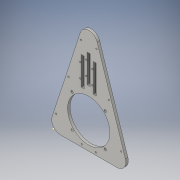
# Autodesk Inventor part: Nathan_LED_Speaker_Front
Saved by Autodesk Inventor 2016 (Build 200138000, 138)
## iProperties
Created: 2018-09-27
Part Number: Nathan_LED_Speaker_Front
Material: Generic
Document SubType Name: Modeling
Designer: Student
Density: 1 g/cm^3
Appearance: Default
Author: Student
Autodesk Inventor part; units mm, degrees
ref_plane "YZ Plane" through (0, 0, 0) normal (1, 0, 0) x (0, 1, 0)
ref_plane "XZ Plane" through (0, 0, 0) normal (0, 1, 0) x (-1, 0, 0)
ref_plane "XY Plane" through (0, 0, 0) normal (0, 0, 1) x (1, 0, 0)
sketch "Sketch1" plane through (0, 0, 0) normal (0, 0, 1) x (1, 0, 0)
  line L0 (63.5, 50.8) -> (63.5, 44.45)
  circle A0 centre (63.5, 44.45) radius 38.1
  circle A1 centre (33.655, 74.295) radius 2.1082
  circle A2 centre (93.345, 74.295) radius 2.1082
  circle A3 centre (93.345, 14.605) radius 2.1082
  circle A4 centre (33.655, 14.605) radius 2.1082
  line L1 (63.5, 82.55) -> (63.5, 86.36)
  line L2 (63.5, 86.36) -> (82.55, 86.36)
  line L3 (63.5, 86.36) -> (44.45, 86.36)
  line L4 (82.55, 86.36) -> (82.55, 134.62)
  line L5 (44.45, 86.36) -> (44.45, 134.62)
  arc A5 (82.55, 134.62) -> (44.45, 134.62) centre (63.5, 134.62) ccw
  arc A6 (-2.400661, 17.597517) -> (12.7, -3.175) centre (12.7, 12.7) ccw
  arc A7 (114.3, -3.175) -> (129.400661, 17.597517) centre (114.3, 12.7) ccw
  line L6 (114.3, -3.175) -> (12.7, -3.175)
  line L7 (48.399339, 174.230681) -> (-2.400661, 17.597517)
  line L8 (129.400661, 17.597517) -> (78.600661, 174.230681)
  arc A8 (78.600661, 174.230681) -> (48.399339, 174.230681) centre (63.5, 169.333164) ccw
  arc A9 (75.580529, 173.251177) -> (51.419471, 173.251177) centre (63.5, 169.333164) ccw
  arc A10 (0.619471, 16.618013) -> (12.7, 0) centre (12.7, 12.7) ccw
  arc A11 (114.3, 0) -> (126.380529, 16.618013) centre (114.3, 12.7) ccw
  line L9 (12.7, 0) -> (114.3, 0)
  line L10 (0.619471, 16.618013) -> (51.419471, 173.251177)
  line L11 (75.580529, 173.251177) -> (126.380529, 16.618013)
  line L12 (0.619471, 16.618013) -> (3.753882, 26.282436)
  line L13 (3.753882, 26.282436) -> (4.961935, 25.890635)
  circle A12 centre (4.961935, 25.890635) radius 1.27
  line L14 (51.419471, 173.251177) -> (48.285061, 163.586755)
  line L15 (48.285061, 163.586755) -> (49.493113, 163.194953)
  circle A13 centre (49.493113, 163.194953) radius 1.27
  circle A14 centre (27.227524, 94.542794) radius 1.27
  line L16 (75.580529, 173.251177) -> (78.714939, 163.586755)
  line L17 (78.714939, 163.586755) -> (77.506886, 163.194953)
  circle A15 centre (77.506886, 163.194953) radius 1.27
  line L18 (126.380529, 16.618013) -> (123.246118, 26.282436)
  line L19 (123.246118, 26.282436) -> (122.038065, 25.890635)
  circle A16 centre (122.038065, 25.890635) radius 1.27
  circle A17 centre (99.772476, 94.542794) radius 1.27
  line L20 (12.7, 0) -> (16.51, 0)
  line L21 (18.621315, -3.175) -> (18.621315, 1.27) construction
  line L22 (45.72, 1.27) -> (50.8, 1.27) construction
  line L23 (12.7, 0.808162) -> (16.51, 0.808162) construction
  circle A18 centre (50.8, 1.27) radius 1.27
  line L24 (109.391635, -3.175) -> (109.391635, 1.27) construction
  line L25 (81.28, 1.27) -> (76.2, 1.27) construction
  line L26 (114.432893, 0.578481) -> (110.622893, 0.578481) construction
  circle A19 centre (76.2, 1.27) radius 1.27
  point P0 (0, 0)
  point P1 (0, 0)
  dimension "d13" = 76.2
  dimension "d42" = 2.54
  dimension "d45" = 2.54
  dimension "d12" = 6.35
  dimension "d14" = 4.2164
  dimension "d15" = 4.2164
  dimension "d16" = 4.2164
  dimension "d17" = 4.2164
  dimension "d18" = 3.81
  dimension "d19" = 19.05
  dimension "d20" = 19.05
  dimension "d21" = 48.26
  dimension "d22" = 48.26
  dimension "d26" = 31.75
  dimension "d27" = 31.75
  dimension "d30" = 25.4
  dimension "d31" = 25.4
  dimension "d32" = 25.4
  dimension "d33" = 10.16
  dimension "d34" = 10.16
  dimension "d35" = 1.27
  dimension "d37" = 1.27
  dimension "d40" = 10.16
  dimension "d41" = 10.16
  dimension "d43" = 2.54
  dimension "d44" = 2.54
  dimension "d221" = 4.445
  dimension "d222" = 5.08
  dimension "d224" = 5.08
  dimension "d225" = 3.81
  dimension "d228" = 38.1
  dimension "d229" = 38.1
  constraints: 54 end point, 15 centre point, 14 point on circle, 10 coincident, 7 point on line, 6 horizontal, 6 tangent, 6 vertical, 1 perpendicular, 1 vertical alignment, 14 other
  measures "d12" distance of L0.start L0.end
  measures "d14" diameter of A1
  measures "d15" diameter of A2
  measures "d16" diameter of A3
  measures "d17" diameter of A4
  measures "d18" distance of L1.start L1.end
  measures "d19" distance of L1.end L2.end
  measures "d20" distance of L1.end L3.end
  measures "d21" distance of L2.end L4.end
  measures "d22" distance of L3.end L5.end
  measures "d26" diameter of A6
  measures "d27" diameter of A7
  measures "d30" diameter of A9
  measures "d31" diameter of A10
  measures "d32" diameter of A11
  measures "d33" distance of L10.start L12.end
  measures "d34" distance of L10.end L14.end
  measures "d35" distance of L14.end L15.end
  measures "d37" distance of L16.end L17.end
  measures "d40" distance of L11.end L18.end
  measures "d41" distance of L16.end L11.start
  measures "d43" diameter of A14
  measures "d44" diameter of A17
  measures "d221" distance of L21.start L21.end
  measures "d222" distance of L22.start L22.end
  measures "d224" distance of L25.start L25.end
  measures "d225" distance of L26.start L26.end
  measures "d228" horizontal distance of L25.end L6.start
  measures "d229" horizontal distance of L22.end L6.end
sketch "Sketch1 outline for Extrusion3" plane through (0, 0, 0) normal (0, 0, 1) x (1, 0, 0)
  arc A0 (78.600661, 174.230681) -> (48.399339, 174.230681) centre (63.5, 169.333164) ccw
  line L0 (129.400661, 17.597517) -> (78.600661, 174.230681)
  line L1 (48.399339, 174.230681) -> (-2.400661, 17.597517)
  arc A1 (114.3, -3.175) -> (129.400661, 17.597517) centre (114.3, 12.7) ccw
  arc A2 (-2.400661, 17.597517) -> (12.7, -3.175) centre (12.7, 12.7) ccw
  line L2 (12.7, -3.175) -> (114.3, -3.175)
  circle A3 centre (4.961935, 25.890635) radius 1.27
  circle A4 centre (33.655, 14.605) radius 2.1082
  circle A5 centre (33.655, 74.295) radius 2.1082
  circle A6 centre (93.345, 14.605) radius 2.1082
  circle A7 centre (63.5, 44.45) radius 38.1
  circle A8 centre (122.038065, 25.890635) radius 1.27
  circle A9 centre (93.345, 74.295) radius 2.1082
  circle A10 centre (27.227524, 94.542794) radius 1.27
  circle A11 centre (49.493113, 163.194953) radius 1.27
  line L3 (44.45, 86.36) -> (63.5, 86.36)
  line L4 (63.5, 86.36) -> (82.55, 86.36)
  line L5 (82.55, 86.36) -> (82.55, 134.62)
  arc A12 (82.55, 134.62) -> (44.45, 134.62) centre (63.5, 134.62) ccw
  line L6 (44.45, 134.62) -> (44.45, 86.36)
  circle A13 centre (99.772476, 94.542794) radius 1.27
  circle A14 centre (77.506886, 163.194953) radius 1.27
extrude "Extrusion3" add sketch "Sketch1 outline for Extrusion3" along normal blind 4.572
sketch "Sketch2" plane through (0, 0, 4.572) normal (0, 0, 1) x (1, 0, 0)
  line L0 (44.45, 86.36) -> (82.55, 86.36)
  line L1 (63.5, 86.36) -> (44.45, 86.36)
  line L2 (63.5, 86.36) -> (82.55, 86.36)
  line L3 (53.975, 86.36) -> (63.5, 86.36)
  line L4 (63.5, 86.36) -> (73.025, 86.36)
  line L5 (82.55, 134.62) -> (82.55, 86.36)
  line L6 (71.882, 140.7922) -> (76.962, 140.7922)
  line L7 (76.962, 140.7922) -> (76.962, 89.9922)
  line L8 (76.962, 89.9922) -> (71.882, 89.9922)
  line L9 (71.882, 89.9922) -> (71.882, 140.7922)
  circle A0 centre (70.07225, 128.0922) radius 1.3335
  circle A1 centre (70.07225, 102.6922) radius 1.3335
  line L10 (50.038, 89.9922) -> (55.118, 89.9922)
  line L11 (55.118, 89.9922) -> (55.118, 140.7922)
  line L12 (55.118, 140.7922) -> (50.038, 140.7922)
  line L13 (50.038, 140.7922) -> (50.038, 89.9922)
  line L14 (44.45, 86.36) -> (44.45, 134.62)
  circle A2 centre (48.22825, 128.0922) radius 1.3335
  circle A3 centre (48.22825, 102.6922) radius 1.3335
  line L15 (71.882, 99.06) -> (68.73875, 99.06)
  line L16 (66.04, 99.06) -> (60.96, 99.06)
  line L17 (60.96, 99.06) -> (60.96, 149.86)
  line L18 (60.96, 149.86) -> (66.04, 149.86)
  line L19 (66.04, 149.86) -> (66.04, 99.06)
  circle A4 centre (59.15025, 111.76) radius 1.3335
  circle A5 centre (59.15025, 137.16) radius 1.3335
  arc A6 (82.55, 134.62) -> (44.45, 134.62) centre (63.5, 134.62) ccw
  line L20 (44.45, 134.62) -> (44.45, 86.36)
  point P0 (0, 0)
  dimension "d183" = 5.08
  dimension "d184" = 50.8
  dimension "d185" = 3.6322
  dimension "d186" = 5.588
  dimension "d189" = 2.667
  dimension "d194" = 5.08
  dimension "d196" = 3.6322
  dimension "d197" = 5.588
  dimension "d198" = 50.8
  dimension "d199" = 1.80975
  dimension "d203" = 2.667
  dimension "d204" = 2.667
  dimension "d205" = 1.80975
  dimension "d207" = 41.7322
  dimension "d208" = 16.3322
  dimension "d209" = 1.80975
  dimension "d211" = 5.08
  dimension "d212" = 50.8
  dimension "d216" = 2.667
  dimension "d217" = 2.667
  constraints: 39 end point, 7 centre point, 6 horizontal, 6 parallel, 3 collinear, 3 midpoint, 3 perpendicular, 2 point on circle, 2 point on line, 1 vertical
  measures "d183" distance of L7.end L8.end
  measures "d184" distance of L6.end L7.end
  measures "d185" distance between parallel lines of L2 L8
  measures "d186" distance between parallel lines of L5 L7
  measures "d189" diameter of A0
  measures "d194" distance of L12.end L11.end
  measures "d196" distance between parallel lines of L1 L10
  measures "d197" distance between parallel lines of L14 L13
  measures "d198" distance of L12.end L10.start
  measures "d199" distance from line of L9 A1.centre
  measures "d203" diameter of A2
  measures "d204" diameter of A3
  measures "d205" distance from line of L13 A2.centre
  measures "d207" distance from line of L0 A2.centre
  measures "d208" distance from line of L0 A3.centre
  measures "d209" distance from line of L13 A3.centre
  measures "d211" distance of L17.end L18.end
  measures "d212" distance of L16.end L17.end
  measures "d216" diameter of A4
  measures "d217" diameter of A5
extrude "Extrusion11" add sketch "Sketch2" against normal blind 4.572
sketch "Sketch3" plane through (0, 0, 4.572) normal (0, 0, 1) x (1, 0, 0)
  point P0 (0, 0)
sketch "Sketch1 outline for Extrusion12" plane through (0, 0, 0) normal (0, 0, 1) x (1, 0, 0)
  circle A0 centre (50.8, 1.27) radius 1.27
  circle A1 centre (76.2, 1.27) radius 1.27
extrude "Extrusion12" cut sketch "Sketch1 outline for Extrusion12" along normal blind 4.572
body "Solid3"
